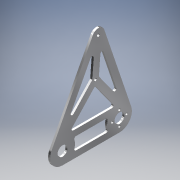
# Autodesk Inventor part: Module Plate
Saved by Autodesk Inventor 2019.4 (Build 234330000, 330)
## iProperties
Created: 2019-12-31
Part Number: Module Plate
Material: Aluminum 6061
Document SubType Name: Modeling
Designer: Mark
Mass: 280.301 g
Surface Area: 508.362 cm^2
Volume: 103.815 cm^3
Density: 2.7 g/cm^3
Appearance: Aluminum - Flat
Author: Mark
Autodesk Inventor part; units mm, degrees
ref_plane "YZ Plane" through (0, 0, 0) normal (1, 0, 0) x (0, 1, 0)
ref_plane "XZ Plane" through (0, 0, 0) normal (0, 1, 0) x (-1, 0, 0)
ref_plane "XY Plane" through (0, 0, 0) normal (0, 0, 1) x (1, 0, 0)
sketch "Sketch1" plane through (0, 0, 0) normal (1, 0, 0) x (0, 1, 0)
  circle A0 centre (0, 0) radius 12
  circle A1 centre (0, -137.4) radius 12
  line L0 (0, 0) -> (0, -137.4)
  line L1 (0, 0) -> (137.4, 0) construction
  line L2 (0, 0) -> (0, -137.4) construction
  line L3 (-30, 0) -> (-30, -137.4)
  line L4 (30, -137.4) -> (30, 0)
  arc A2 (30, 0) -> (-30, 0) centre (0, 0) ccw
  arc A3 (-30, -137.4) -> (30, -137.4) centre (0, -137.4) ccw
  circle A4 centre (0, -137.4) radius 17.5 construction
  line L5 (0, -137.4) -> (17.5, -137.4) construction
  line L6 (0, -137.4) -> (17.5, -137.4) construction
  circle A5 centre (17.5, -137.4) radius 2.65
  line L7 (0, -137.4) -> (0, -119.9) construction
  circle A6 centre (0, -119.9) radius 2.65
  line L8 (0, -137.4) -> (-17.5, -137.4) construction
  circle A7 centre (-17.5, -137.4) radius 2.65
  line L9 (0, -137.4) -> (0, -154.9) construction
  circle A8 centre (0, -154.9) radius 2.65
  line L10 (0, -137.4) -> (198.7323, -86.42) construction
  line L11 (0, -137.4) -> (205.167, -137.4) construction
  circle A9 centre (198.7323, -86.42) radius 5.1
  arc A10 (203.5118, -100.6382) -> (205.6519, -73.1113) centre (198.7323, -86.42) ccw
  line L12 (203.5118, -100.6382) -> (9.559, -165.8363)
  line L13 (205.6519, -73.1113) -> (13.839, 26.6173)
  circle A11 centre (99.5809, 178.6423) radius 283 construction
  circle A12 centre (99.5809, 178.6423) radius 233 construction
  circle A13 centre (0, -137.4) radius 205.167 construction
  line L14 (0, -137.4) -> (198.7323, -86.42) construction
  line L15 (0, -137.4) -> (180.496, -39.8566) construction
  circle A14 centre (99.5809, 178.6423) radius 5 projected
  point P0 (0, -68.7)
  point P1 (-20.8357, -21.5841)
  dimension "d9" = 35
  dimension "d23" = 566
  dimension "d31" = 466
  dimension "d0" = 24
  dimension "d1" = 24
  dimension "d4" = 90
  dimension "d5" = 137.4
  dimension "d6" = 60
  dimension "d10" = 0
  dimension "d11" = 5.3
  dimension "d14" = 360
  dimension "d18" = 10.2
  dimension "d19" = 30
  dimension "d27" = 14
  constraints: 34 end point, 11 centre point, 11 point on circle, 8 tangent, 6 coincident, 3 equal length, 3 horizontal, 2 vertical, 1 horizontal alignment, 1 midpoint, 1 parallel, 30 other
  measures "d0" diameter of A0
  measures "d1" diameter of A1
  measures "d4" angle of L0 L1
  measures "d5" distance of L0.start L0.end
  measures "d6" diameter of A3
  measures "d10" distance between parallel lines of L5 L6
  measures "d11" diameter of A5
  measures "d18" diameter of A9
  measures "d19" diameter of A10
  measures "d27" angle of L14 L15
extrude "Extrusion1" add sketch "Sketch1" along normal blind 5 contours A2 L4 A3 L3 | L13 A10 L12 A3 L4 A2 | A9
sketch "Sketch2" plane through (5, 0, 0) normal (1, 0, 0) x (0, 0, -1)
  circle A0 centre (86.42, 198.7323) radius 3.25
  arc A1 (100.6382, 203.5118) -> (73.1113, 205.6519) centre (86.42, 198.7323) ccw projected
  point P0 (0, 0)
  point P1 (17.6579, 112.2275)
  dimension "d20" = 6.5
  constraints: 1 centre point, 2 other
  measures "d20" diameter of A0
extrude "Extrusion2" cut sketch "Sketch2" against normal blind 10
sketch "Sketch4" plane through (0, 0, 0) normal (-1, 0, 0) x (0, 0, 1)
  line L0 (-92.2196, 178.3412) -> (-138.5391, 40.5491)
  line L1 (-130.956, 30) -> (-12.9947, 30)
  line L2 (-5.8968, 41.6904) -> (-77.5386, 179.4826)
  line L3 (-73.1113, 205.6519) -> (26.6173, 13.839) projected
  line L4 (-165.8363, 9.559) -> (-100.6382, 203.5118) projected
  line L5 (0, -30) -> (-137.4, -30) projected
  arc A0 (-77.5386, 179.4826) -> (-92.2196, 178.3412) centre (-84.6365, 175.7921) ccw
  arc A1 (-138.5391, 40.5491) -> (-130.956, 30) centre (-130.956, 38) ccw
  arc A2 (-12.9947, 30) -> (-5.8968, 41.6904) centre (-12.9947, 38) ccw
  arc A3 (-25.9808, 15) -> (-25.9808, -15) centre (0, 0) ccw
  arc A4 (-111.4192, -15) -> (-111.4192, 15) centre (-137.4, 0) ccw
  line L6 (-111.4192, 15) -> (-25.9808, 15)
  line L7 (-25.9808, -15) -> (-111.4192, -15)
  circle A5 centre (0, 0) radius 12 projected
  circle A6 centre (-137.4, 0) radius 12 projected
  circle A7 centre (-8.3957, 63.839) radius 3.25
  circle A8 centre (-56, -22.5) radius 3.25
  dimension "d38" = 16
  dimension "d39" = 16
  dimension "d40" = 60
  dimension "d41" = 8
  dimension "d42" = 8
  dimension "d43" = 8
  dimension "d69" = 30
  dimension "d70" = 30
  dimension "d71" = 30
  dimension "d72" = 15
  dimension "d82" = 6.5
  dimension "d83" = 6.5
  dimension "d84" = 8
  dimension "d85" = 50
  dimension "d86" = 7.5
  dimension "d87" = 56
  constraints: 10 end point, 10 point on circle, 7 centre point, 6 tangent, 4 parallel, 2 concentric, 1 horizontal
  measures "d38" distance between parallel lines of L3 L2
  measures "d39" distance between parallel lines of L4 L0
  measures "d40" distance between parallel lines of L5 L1
  measures "d41" radius of A0
  measures "d42" radius of A1
  measures "d43" radius of A2
  measures "d69" radius of A3
  measures "d70" radius of A4
  measures "d71" distance between parallel lines of L6 L7
  measures "d72" distance between parallel lines of L5 L7
  measures "d82" diameter of A7
  measures "d83" diameter of A8
  measures "d84" distance from line of L3 A7.centre
  measures "d85" vertical distance of L3.end A7.centre
  measures "d86" distance from line of L5 A8.centre
  measures "d87" horizontal distance of L5.start A8.centre
extrude "Extrusion3" cut sketch "Sketch4" against normal blind 10 contours A0 L2 A2 L1 A1 L0 | A3 L7 A4 L6 | A7 | A8
sketch "Sketch5" plane through (0, 0, 0) normal (-1, 0, 0) x (0, 0, 1)
  circle A0 centre (-79.4844, 109.5205) radius 3.25
  circle A1 centre (-79.4844, 109.5205) radius 8
  line L0 (-73.1113, 205.6519) -> (26.6173, 13.839) projected
  line L1 (-165.8363, 9.559) -> (-100.6382, 203.5118) projected
  line L2 (-79.4844, 109.5205) -> (-130.956, 38) construction
  line L3 (-85.9777, 114.1936) -> (-137.4493, 42.6731)
  line L4 (-124.4628, 33.3269) -> (-72.9911, 104.8475)
  arc A2 (-72.9911, 104.8475) -> (-85.9777, 114.1936) centre (-79.4844, 109.5205) ccw
  arc A3 (-137.4493, 42.6731) -> (-124.4628, 33.3269) centre (-130.956, 38) ccw
  line L5 (-79.4844, 109.5205) -> (-12.9947, 38) construction
  line L6 (-85.3436, 104.0735) -> (-18.8539, 32.553)
  line L7 (-7.1355, 43.447) -> (-73.6252, 114.9675)
  arc A4 (-73.6252, 114.9675) -> (-85.3436, 104.0735) centre (-79.4844, 109.5205) ccw
  arc A5 (-18.8539, 32.553) -> (-7.1355, 43.447) centre (-12.9947, 38) ccw
  arc A6 (-12.9947, 30) -> (-5.8968, 41.6904) centre (-12.9947, 38) ccw projected
  line L8 (-79.4844, 109.5205) -> (-84.6365, 175.7921) construction
  line L9 (-71.5085, 110.1406) -> (-76.6606, 176.4122)
  line L10 (-92.6125, 175.1721) -> (-87.4603, 108.9004)
  arc A7 (-87.4603, 108.9004) -> (-71.5085, 110.1406) centre (-79.4844, 109.5205) ccw
  arc A8 (-76.6606, 176.4122) -> (-92.6125, 175.1721) centre (-84.6365, 175.7921) ccw
  arc A9 (-77.5386, 179.4826) -> (-92.2196, 178.3412) centre (-84.6365, 175.7921) ccw projected
  arc A10 (-138.5391, 40.5491) -> (-130.956, 30) centre (-130.956, 38) ccw projected
  line L11 (-75.8855, 166.4423) -> (-91.8374, 165.2022)
  line L12 (-91.8374, 165.2022) -> (-93.3876, 185.142)
  line L13 (-93.3876, 185.142) -> (-77.4357, 186.3821)
  line L14 (-77.4357, 186.3821) -> (-75.8855, 166.4423)
  line L15 (-75.8855, 166.4423) -> (-93.3876, 185.142) construction
  line L16 (-91.8374, 165.2022) -> (-77.4357, 186.3821) construction
  line L17 (-25.6627, 39.8769) -> (-13.9443, 50.771)
  line L18 (-13.9443, 50.771) -> (-0.3267, 36.1231)
  line L19 (-0.3267, 36.1231) -> (-12.0451, 25.229)
  line L20 (-12.0451, 25.229) -> (-25.6627, 39.8769)
  line L21 (-25.6627, 39.8769) -> (-0.3267, 36.1231) construction
  line L22 (-13.9443, 50.771) -> (-12.0451, 25.229) construction
  line L23 (-131.608, 50.7896) -> (-118.6215, 41.4435)
  line L24 (-118.6215, 41.4435) -> (-130.3041, 25.2104)
  line L25 (-130.3041, 25.2104) -> (-143.2906, 34.5565)
  line L26 (-143.2906, 34.5565) -> (-131.608, 50.7896)
  line L27 (-131.608, 50.7896) -> (-130.3041, 25.2104) construction
  line L28 (-118.6215, 41.4435) -> (-143.2906, 34.5565) construction
  circle A11 centre (-137.4, 0) radius 12 projected
  arc A12 (-25.9808, 15) -> (-25.9808, -15) centre (0, 0) ccw
  arc A13 (-111.4192, -15) -> (-111.4192, 15) centre (-137.4, 0) ccw
  circle A14 centre (0, 0) radius 12 projected
  line L29 (-111.4192, 15) -> (-25.9808, 15)
  line L30 (-25.9808, -15) -> (-111.4192, -15)
  line L31 (0, -30) -> (-137.4, -30) projected
  circle A15 centre (-8.3957, 63.839) radius 3.25
  circle A16 centre (-8.3957, 63.839) radius 5 construction
  circle A17 centre (-56.5, -22.5) radius 5 construction
  circle A18 centre (-56.5, -22.5) radius 3.25
  point P0 (-105.2202, 73.7603)
  point P1 (-46.2395, 73.7603)
  point P2 (-82.0605, 142.6563)
  dimension "d46" = 6.5
  dimension "d47" = 16
  dimension "d48" = 50
  dimension "d49" = 50
  dimension "d50" = 16
  dimension "d51" = 16
  dimension "d52" = 16
  dimension "d55" = 20
  dimension "d56" = 90
  dimension "d57" = 20
  dimension "d58" = 20
  dimension "d65" = 30
  dimension "d66" = 30
  dimension "d67" = 30
  dimension "d68" = 15
  dimension "d74" = 6.5
  dimension "d75" = 10
  dimension "d76" = 8
  dimension "d77" = 50
  dimension "d78" = 10
  dimension "d79" = 7.5
  dimension "d80" = 6.5
  dimension "d81" = 56.5
  constraints: 65 end point, 16 point on circle, 14 centre point, 12 tangent, 10 parallel, 9 midpoint, 5 concentric, 5 perpendicular, 3 coincident, 1 horizontal
  measures "d46" diameter of A0
  measures "d47" diameter of A1
  measures "d48" distance from line of L0 L2.start
  measures "d49" distance from line of L1 L2.start
  measures "d50" diameter of A3
  measures "d51" diameter of A5
  measures "d52" diameter of A8
  measures "d55" distance of L11.end L12.end
  measures "d56" angle of L9 L11
  measures "d57" distance of L17.end L18.end
  measures "d58" distance of L23.end L24.end
  measures "d65" radius of A12
  measures "d66" radius of A13
  measures "d67" distance between parallel lines of L29 L30
  measures "d68" distance between parallel lines of L31 L30
  measures "d74" diameter of A15
  measures "d75" diameter of A16
  measures "d76" distance from line of L0 A16.centre
  measures "d77" vertical distance of L0.end A15.centre
  measures "d78" diameter of A17
  measures "d79" distance from line of L30 A17.centre
  measures "d80" diameter of A18
  measures "d81" horizontal distance of L31.start A18.centre
extrude "Extrusion4" add sketch "Sketch5" against normal blind 5 contours A1 | A1 L9 L7 L17 L6 L4 | A1 L7 L9 | L4 L6 A1 | A1 L3 L10 L11 L9 L7 | L6 L4 L23 L3 L10 A1 | A1 L10 L3 | L7 A5 L6 L17 | L11 L10 A8 L9 | L4 A3 L3 L23 | L18 L19 L20 A5 | A8 L12 L13 L14 | L24 L25 L26 A3
fillet "Fillet1" radius 4 13 edges at (2.5, 30, -126.8571) (2.5, 41.6933, -138.1544) (2.5, 176.7967, -92.7388) (2.5, 111.8182, -87.6872) (2.5, 112.9233, -71.7248) (2.5, 96.9219, -78.695) (2.5, 178.0368, -76.7869) (2.5, 42.6527, -6.3971) (2.5, 30, -16.4805) (2.5, 15, -111.4192) (2.5, -15, -111.4192) (2.5, 15, -25.9808) (2.5, -15, -25.9808)
body "Solid1"
